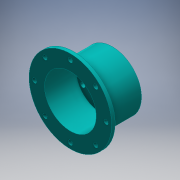
# Autodesk Inventor part: motor fixture
Saved by Autodesk Inventor 2016 (Build 200138000, 138)
## iProperties
Created: 2016-06-30
Part Number: motor fixture
Material: ABS Plastic
Document SubType Name: Modeling
Designer: hesaon
Density: 1.06 g/cm^3
Appearance: Smooth - White
Author: hesaon
Autodesk Inventor part; units mm, degrees
ref_plane "YZ Plane" through (0, 0, 0) normal (1, 0, 0) x (0, 1, 0)
ref_plane "XZ Plane" through (0, 0, 0) normal (0, 1, 0) x (-1, 0, 0)
ref_plane "XY Plane" through (0, 0, 0) normal (0, 0, 1) x (1, 0, 0)
sketch "Sketch2" plane through (0, 0, 0) normal (0, 1, 0) x (-1, 0, 0)
  circle A0 centre (0, 0) radius 18.75
  circle A1 centre (0, 0) radius 30
  circle A2 centre (26, 0) radius 1.6
  circle A3 centre (18.3848, -18.3848) radius 1.6
  circle A4 centre (0, -26) radius 1.6
  circle A5 centre (-18.3848, -18.3848) radius 1.6
  circle A6 centre (-26, 0) radius 1.6
  circle A7 centre (-18.3848, 18.3848) radius 1.6
  circle A8 centre (0, 26) radius 1.6
  circle A9 centre (18.3848, 18.3848) radius 1.6
  dimension "motorDiameter" = 37.5
  dimension "motorFixtureDiameter" = 60
  dimension "d20" = 3.2
  dimension "d21" = 26
  dimension "d24" = 0
  dimension "d27" = 360
  constraints: 10 centre point, 2 coincident, 17 other
  measures "motorDiameter" diameter of A0
  measures "motorFixtureDiameter" diameter of A1
  measures "d20" diameter of A2
  measures "d21" distance of point (0, 0) A2.centre
  measures "d24" vertical distance of point (0, 0) A2.centre
extrude "Extrusion2" add sketch "Sketch2" along normal blind 2.5
sketch "Sketch3" plane through (0, 2.5, 0) normal (0, 1, 0) x (1, 0, 0)
  circle A0 centre (2, 0) radius 21.15
  circle A1 centre (0, 0) radius 18.75
  dimension "d31" = 2
  dimension "d32" = 42.3
  dimension "d33" = 37.5
  dimension "d34" = 0
  constraints: 2 centre point, 1 coincident
  measures "d31" distance of point (0, 0) A0.centre
  measures "d32" diameter of A0
  measures "d33" diameter of A1
  measures "d34" vertical distance of point (0, 0) A0.centre
extrude "Extrusion3" add sketch "Sketch3" along normal blind 20
sketch "Sketch4" plane through (2, 22.5, 0) normal (0, 1, 0) x (1, 0, 0)
  circle A0 centre (0, 0) radius 21.15 projected
  circle A1 centre (0, 0) radius 21.15
  constraints: 1 centre point, 1 coincident
extrude "Extrusion4" add sketch "Sketch4" along normal blind 6
sketch "Sketch5" plane through (2, 28.5, 0) normal (0, 1, 0) x (1, 0, 0)
  circle A0 centre (-2, 0) radius 18.75 projected
  circle A1 centre (0, 0) radius 21.15 projected
  circle A2 centre (0, 0) radius 21.15 projected
  circle A3 centre (5, 0) radius 6.25
  circle A4 centre (-2, 15.5) radius 1.6
  circle A5 centre (-15.4234, 7.75) radius 1.6
  circle A6 centre (-15.4234, -7.75) radius 1.6
  circle A7 centre (-2, -15.5) radius 1.6
  circle A8 centre (11.4234, -7.75) radius 1.6
  circle A9 centre (11.4234, 7.75) radius 1.6
  dimension "d39" = 12.5
  dimension "d40" = 0
  dimension "d43" = 3.2
  dimension "d44" = 0
  dimension "d45" = 15.5
  dimension "d48" = 360
  dimension "d52" = 7
  constraints: 7 centre point, 13 other
  measures "d39" diameter of A3
  measures "d40" vertical distance of A1.centre A3.centre
  measures "d43" diameter of A4
  measures "d44" horizontal distance of point (-2, 0) A4.centre
  measures "d45" distance of point (-2, 0) A4.centre
  measures "d52" distance of point (-2, 0) A3.centre
extrude "Extrusion5" cut sketch "Sketch5" against normal up to next contours A3 | A4 | A5 | A6 | A7 | A8 | A9
equation "\"d33\" = motorDiameter"
body "Solid2"
